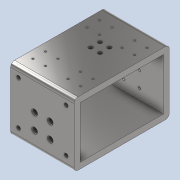
# Autodesk Inventor part: 4in x 6in Steel Rectangular Tubing 4in long
Saved by Autodesk Inventor 2022 (Build 260153000, 153)
## iProperties
Created: 2021-10-11
Part Number: 4in x 6in Steel Rectangular Tubing 4in long
Material: Generic
Document SubType Name: Modeling
Designer: Coy
Density: 1 g/cm^3
Appearance: Galvanized
Author: Coy
Autodesk Inventor part; units mm, degrees
ref_plane "YZ Plane" through (0, 0, 0) normal (1, 0, 0) x (0, 1, 0)
ref_plane "XZ Plane" through (0, 0, 0) normal (0, 1, 0) x (-1, 0, 0)
ref_plane "XY Plane" through (0, 0, 0) normal (0, 0, 1) x (1, 0, 0)
sketch "Sketch1" plane through (0, 0, 0) normal (1, 0, 0) x (0, 1, 0)
  line L0 (6.35, 0) -> (95.25, 0)
  line L1 (101.6, -6.35) -> (101.6, -146.05)
  line L2 (95.25, -152.4) -> (6.35, -152.4)
  line L3 (0, -146.05) -> (0, -6.35)
  arc A0 (101.6, -6.35) -> (95.25, 0) centre (95.25, -6.35) ccw
  arc A1 (95.25, -152.4) -> (101.6, -146.05) centre (95.25, -146.05) ccw
  arc A2 (0, -146.05) -> (6.35, -152.4) centre (6.35, -146.05) ccw
  arc A3 (6.35, 0) -> (0, -6.35) centre (6.35, -6.35) ccw
  line L4 (92.075, -142.875) -> (92.075, -9.525)
  line L5 (92.075, -9.525) -> (9.525, -9.525)
  line L6 (9.525, -9.525) -> (9.525, -142.875)
  line L7 (9.525, -142.875) -> (92.075, -142.875)
  point P0 (0, 0)
  point P1 (101.6, -152.4)
  point P2 (101.6, 0)
  point P3 (0, -152.4)
  dimension "d0" = 101.6
  dimension "d1" = 152.4
  dimension "d2" = 6.35
  dimension "d3" = 6.35
  dimension "d4" = 9.525
  constraints: 16 end point, 8 point on circle, 8 point on line, 8 tangent, 4 centre point, 4 parallel, 2 equal radius, 2 perpendicular, 1 horizontal, 3 other
  measures "d0" distance of point (101.6, -152.4) point (0, -152.4)
  measures "d1" distance of point (101.6, 0) point (101.6, -152.4)
  measures "d2" radius of A0
  measures "d3" radius of A3
  measures "d4" distance between parallel lines of L1 L4
extrude "Extrusion1" add sketch "Sketch1" against normal blind 101.6
sketch "Sketch2" plane through (0, 101.6, -6.35) normal (0, 1, 0) x (1, 0, 0)
  line L0 (0, 0) -> (0, 139.7) construction
  line L1 (0, 69.85) -> (-101.6, 69.85) construction
  line L2 (-101.6, 139.7) -> (-101.6, 0) construction
  line L3 (0, 99.6) -> (-45.4, 99.6) construction
  line L4 (-45.4, 99.6) -> (-45.4, 126.6) construction
  line L5 (-45.4, 126.6) -> (0, 126.6) construction
  line L6 (0, 126.6) -> (0, 99.6) construction
  line L7 (-32.7, 123.1) -> (-12.7, 123.1) construction
  line L8 (-12.7, 123.1) -> (-12.7, 103.1) construction
  line L9 (-12.7, 103.1) -> (-32.7, 103.1) construction
  line L10 (-32.7, 103.1) -> (-32.7, 123.1) construction
  line L11 (-32.7, 123.1) -> (-32.7, 126.6) construction
  line L12 (-32.7, 123.1) -> (-45.4, 123.1) construction
  line L13 (-12.7, 103.1) -> (-12.7, 99.6) construction
  line L14 (-12.7, 103.1) -> (0, 103.1) construction
  circle A0 centre (-32.7, 123.1) radius 1.6
  circle A1 centre (-12.7, 123.1) radius 1.6
  circle A2 centre (-12.7, 103.1) radius 1.6
  circle A3 centre (-32.7, 103.1) radius 1.6
  line L15 (0, 139.7) -> (0, 0) construction
  line L16 (-50.8, 69.85) -> (-50.8, 128.3257) construction
  line L17 (-101.6, 99.6) -> (-56.2, 99.6) construction
  line L18 (-56.2, 99.6) -> (-56.2, 126.6) construction
  line L19 (-56.2, 126.6) -> (-101.6, 126.6) construction
  line L20 (-101.6, 126.6) -> (-101.6, 99.6) construction
  line L21 (-68.9, 123.1) -> (-88.9, 123.1) construction
  line L22 (-88.9, 123.1) -> (-88.9, 103.1) construction
  line L23 (-88.9, 103.1) -> (-68.9, 103.1) construction
  line L24 (-68.9, 103.1) -> (-68.9, 123.1) construction
  line L25 (-68.9, 123.1) -> (-68.9, 126.6) construction
  line L26 (-68.9, 123.1) -> (-56.2, 123.1) construction
  line L27 (-88.9, 103.1) -> (-88.9, 99.6) construction
  line L28 (-88.9, 103.1) -> (-101.6, 103.1) construction
  circle A4 centre (-68.9, 123.1) radius 1.6
  circle A5 centre (-88.9, 123.1) radius 1.6
  circle A6 centre (-88.9, 103.1) radius 1.6
  circle A7 centre (-68.9, 103.1) radius 1.6
  line L29 (0, 40.1) -> (-45.4, 40.1) construction
  line L30 (-45.4, 40.1) -> (-45.4, 13.1) construction
  line L31 (-45.4, 13.1) -> (0, 13.1) construction
  line L32 (0, 13.1) -> (0, 40.1) construction
  line L33 (-32.7, 16.6) -> (-12.7, 16.6) construction
  line L34 (-12.7, 16.6) -> (-12.7, 36.6) construction
  line L35 (-12.7, 36.6) -> (-32.7, 36.6) construction
  line L36 (-32.7, 36.6) -> (-32.7, 16.6) construction
  line L37 (-32.7, 16.6) -> (-32.7, 13.1) construction
  line L38 (-32.7, 16.6) -> (-45.4, 16.6) construction
  line L39 (-12.7, 36.6) -> (-12.7, 40.1) construction
  line L40 (-12.7, 36.6) -> (0, 36.6) construction
  circle A8 centre (-32.7, 16.6) radius 1.6
  circle A9 centre (-12.7, 16.6) radius 1.6
  circle A10 centre (-12.7, 36.6) radius 1.6
  circle A11 centre (-32.7, 36.6) radius 1.6
  line L41 (-68.9, 16.6) -> (-88.9, 16.6) construction
  line L42 (-88.9, 36.6) -> (-68.9, 36.6) construction
  line L43 (-88.9, 36.6) -> (-88.9, 40.1) construction
  line L44 (-88.9, 16.6) -> (-88.9, 36.6) construction
  circle A12 centre (-88.9, 36.6) radius 1.6
  circle A13 centre (-88.9, 16.6) radius 1.6
  line L45 (-101.6, 40.1) -> (-56.2, 40.1) construction
  line L46 (-101.6, 13.1) -> (-101.6, 40.1) construction
  line L47 (-88.9, 36.6) -> (-101.6, 36.6) construction
  line L48 (-56.2, 13.1) -> (-101.6, 13.1) construction
  line L49 (-68.9, 36.6) -> (-68.9, 16.6) construction
  line L50 (-68.9, 16.6) -> (-68.9, 13.1) construction
  circle A14 centre (-68.9, 16.6) radius 1.6
  circle A15 centre (-68.9, 36.6) radius 1.6
  line L51 (-56.2, 40.1) -> (-56.2, 13.1) construction
  line L52 (-68.9, 16.6) -> (-56.2, 16.6) construction
  point P0 (0, -6.35)
  dimension "d7" = 45.4
  dimension "d8" = 27
  dimension "d9" = 20
  dimension "d10" = 20
  dimension "d11" = 3.2
  dimension "d12" = 3.2
  dimension "d13" = 3.2
  dimension "d14" = 3.2
  dimension "d15" = 106.5
  constraints: 100 end point, 48 symmetric about line, 17 point on line, 16 centre point, 16 coincident, 6 parallel, 6 perpendicular, 3 midpoint, 2 horizontal, 1 vertical, 12 other
  measures "d7" distance of L4.end L5.end
  measures "d8" distance of L3.end L4.end
  measures "d9" distance of L8.end L9.end
  measures "d10" distance of L7.end L8.end
  measures "d11" diameter of A0
  measures "d12" diameter of A1
  measures "d13" diameter of A3
  measures "d14" diameter of A2
  measures "d15" diameter of L7 L1
extrude "Extrusion2" cut sketch "Sketch2" against normal up to next
sketch "Sketch3" plane through (0, 6.35, -152.4) normal (0, 0, -1) x (-1, 0, 0)
  line L0 (38.3, 45.15) -> (63.3, 45.15) construction
  line L1 (63.3, 45.15) -> (63.3, 20.15) construction
  line L2 (63.3, 20.15) -> (38.3, 20.15) construction
  line L3 (38.3, 20.15) -> (38.3, 45.15) construction
  circle A0 centre (38.3, 45.15) radius 2.1
  circle A1 centre (63.3, 45.15) radius 2.1
  circle A2 centre (63.3, 20.15) radius 2.1
  circle A3 centre (38.3, 20.15) radius 2.1
  line L4 (0, -6.35) -> (101.6, -6.35) construction
  line L5 (38.3, 32.65) -> (0, 32.65) construction
  line L6 (0, 0) -> (0, 88.9) construction
  line L7 (63.3, 32.65) -> (101.6, 32.65) construction
  line L8 (101.6, 88.9) -> (101.6, 0) construction
  dimension "d18" = 25
  dimension "d19" = 25
  dimension "d20" = 4.2
  dimension "d21" = 4.2
  dimension "d22" = 4.2
  dimension "d23" = 4.2
  dimension "d24" = 26.5
  constraints: 12 end point, 4 centre point, 4 coincident, 3 horizontal, 2 midpoint, 2 parallel, 2 point on line, 1 collinear, 1 perpendicular
  measures "d18" distance of L1.end L2.end
  measures "d19" distance of L0.end L1.end
  measures "d20" diameter of A0
  measures "d21" diameter of A1
  measures "d22" diameter of A3
  measures "d23" diameter of A2
  measures "d24" distance between parallel lines of L4 L2
extrude "Extrusion3" cut sketch "Sketch3" against normal up to next
sketch "Sketch4" plane through (0, 6.35, 0) normal (0, 0, 1) x (1, 0, 0)
  line L0 (-88.9, 80.5892) -> (-12.7, 80.5892) construction
  line L1 (-12.7, 80.5892) -> (-12.7, 10.7392) construction
  line L2 (-12.7, 10.7392) -> (-88.9, 10.7392) construction
  line L3 (-88.9, 10.7392) -> (-88.9, 80.5892) construction
  line L4 (-88.9, 80.5892) -> (-88.9, 97.6783) construction
  line L5 (-88.9, 80.5892) -> (-101.6, 80.5892) construction
  line L6 (-101.6, 85.725) -> (-101.6, 3.175) construction
  line L7 (-12.7, 10.7392) -> (-12.7, -6.35) construction
  line L8 (0, -6.35) -> (-101.6, -6.35) construction
  line L9 (-12.7, 10.7392) -> (0, 10.7392) construction
  line L10 (0, 85.725) -> (0, 3.175) construction
  circle A0 centre (-12.7, 80.5892) radius 3.175
  circle A1 centre (-12.7, 10.7392) radius 3.175
  circle A2 centre (-88.9, 10.7392) radius 3.175
  circle A3 centre (-88.9, 80.5892) radius 3.175
  circle A4 centre (-63.3, 45.15) radius 2.1 projected
  circle A5 centre (-63.3, 20.15) radius 2.1 projected
  circle A6 centre (-38.3, 45.15) radius 2.1 projected
  circle A7 centre (-38.3, 20.15) radius 2.1 projected
  circle A8 centre (-63.3, 45.15) radius 4.7625
  circle A9 centre (-38.3, 45.15) radius 2.1 projected
  circle A10 centre (-38.3, 45.15) radius 4.7625
  circle A11 centre (-63.3, 20.15) radius 2.1 projected
  circle A12 centre (-63.3, 20.15) radius 4.7625
  circle A13 centre (-38.3, 20.15) radius 2.1 projected
  circle A14 centre (-38.3, 20.15) radius 4.7625
  dimension "d27" = 6.35
  dimension "d28" = 6.35
  dimension "d29" = 6.35
  dimension "d30" = 6.35
  dimension "d31" = 69.85
  dimension "d32" = 76.2
  dimension "d33" = 9.525
  dimension "d34" = 9.525
  dimension "d35" = 9.525
  dimension "d36" = 9.525
  constraints: 16 end point, 8 centre point, 8 coincident, 4 parallel, 3 point on line, 2 horizontal, 2 perpendicular, 2 vertical
  measures "d27" diameter of A0
  measures "d28" diameter of A1
  measures "d29" diameter of A2
  measures "d30" diameter of A3
  measures "d31" distance of L2.end L0.start
  measures "d32" distance of L0.start L0.end
  measures "d33" diameter of A8
  measures "d34" diameter of A10
  measures "d35" diameter of A12
  measures "d36" diameter of A14
extrude "Extrusion4" cut sketch "Sketch4" against normal up to next contours A0 | A1 | A2 | A3 | A4 | A5 | A6 | A7 | A8 | A10 | A12 | A14
thread "Thread1" size "1/4-20 UNC" class "2B" standard "ANSI Unified Screw Threads" full length
thread "Thread2" size "1/4-20 UNC" class "2B" standard "ANSI Unified Screw Threads" full length
thread "Thread3" size "1/4-20 UNC" class "2B" standard "ANSI Unified Screw Threads" full length
thread "Thread4" size "1/4-20 UNC" class "2B" standard "ANSI Unified Screw Threads" full length
sketch "Sketch5" plane through (0, 101.6, -6.35) normal (0, 1, 0) x (1, 0, 0)
  line L0 (21.1594, 98.325) -> (-128.3175, 98.325) construction
  line L1 (0, 146.05) -> (-101.6, 146.05) construction
  circle A0 centre (-32.7, 103.1) radius 1.6 construction
  circle A1 centre (-32.7, 103.1) radius 2.75 construction
  line L2 (0, 3.175) -> (0, 136.525) construction
  line L3 (-101.6, 136.525) -> (-101.6, 3.175) construction
  line L4 (0, 98.325) -> (-101.6, 98.325) construction
  line L5 (-101.6, 98.325) -> (-101.6, 73.325) construction
  line L6 (-101.6, 73.325) -> (0, 73.325) construction
  line L7 (0, 73.325) -> (0, 98.325) construction
  line L8 (-43.3, 78.325) -> (-58.3, 78.325) construction
  line L9 (-58.3, 78.325) -> (-58.3, 93.325) construction
  line L10 (-58.3, 93.325) -> (-43.3, 93.325) construction
  line L11 (-43.3, 93.325) -> (-43.3, 78.325) construction
  line L12 (-43.3, 78.325) -> (0, 78.325) construction
  line L13 (-58.3, 93.325) -> (-101.6, 93.325) construction
  line L14 (-58.3, 93.325) -> (-58.3, 98.325) construction
  line L15 (-43.3, 78.325) -> (-43.3, 73.325) construction
  circle A2 centre (-43.3, 78.325) radius 3.175
  circle A3 centre (-58.3, 78.325) radius 3.175
  circle A4 centre (-58.3, 93.325) radius 3.175
  circle A5 centre (-43.3, 93.325) radius 3.175
  point P0 (0, -6.35)
  dimension "d47" = 47.725
  dimension "d48" = 5.5
  dimension "d49" = 25
  dimension "d50" = 15
  dimension "d51" = 15
  dimension "d52" = 6.35
  dimension "d53" = 6.35
  dimension "d54" = 6.35
  dimension "d55" = 6.35
  constraints: 26 end point, 7 point on line, 6 parallel, 6 perpendicular, 5 centre point, 5 coincident, 3 horizontal
  measures "d47" distance between parallel lines of L1 L0
  measures "d48" diameter of A1
  measures "d49" distance of L5.end L4.end
  measures "d50" distance of L9.end L10.end
  measures "d51" distance of L8.end L9.end
  measures "d52" diameter of A2
  measures "d53" diameter of A3
  measures "d54" diameter of A4
  measures "d55" diameter of A5
extrude "Extrusion5" cut sketch "Sketch5" against normal up to next
thread "Thread5" size "1/4-20 UNC" class "2B" standard "ANSI Unified Screw Threads" full length
thread "Thread6" size "1/4-20 UNC" class "2B" standard "ANSI Unified Screw Threads" full length
thread "Thread7" size "1/4-20 UNC" class "2B" standard "ANSI Unified Screw Threads" full length
thread "Thread8" size "1/4-20 UNC" class "2B" standard "ANSI Unified Screw Threads" full length
equation "\"d12\" = d11"
equation "\"d13\" = d11"
equation "\"d14\" = d11"
equation "\"d16\" = d12"
equation "\"d21\" = d20"
equation "\"d22\" = d20"
equation "\"d23\" = d20"
equation "\"d34\" = d33"
equation "\"d35\" = d33"
equation "\"d36\" = d33"
equation "\"d37\" = d33"
equation "\"d53\" = d52"
equation "\"d54\" = d52"
equation "\"d55\" = d52"
body "Solid1"
